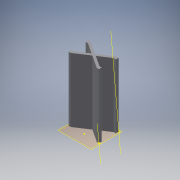
# Autodesk Inventor part: Part3
Saved by Autodesk Inventor 2018 (Build 220112000, 112)
## iProperties
Created: 2019-11-06
Part Number: Part3
Material: Generic
Document SubType Name: Modeling
Designer: bitbots
Density: 1 g/cm^3
Appearance: Default
Author: bitbots
Autodesk Inventor part; units mm, degrees
ref_plane "YZ Plane" through (0, 0, 0) normal (1, 0, 0) x (0, 1, 0)
ref_plane "XZ Plane" through (0, 0, 0) normal (0, 1, 0) x (-1, 0, 0)
ref_plane "XY Plane" through (0, 0, 0) normal (0, 0, 1) x (1, 0, 0)
sketch "Sketch1" plane through (0, 0, 0) normal (0, 0, 1) x (1, 0, 0)
  line L0 (25.85, -1.5771) -> (25.85, -14.5436) construction
  line L1 (25.85, 20.3743) -> (25.85, 33.3441) construction
  line L2 (-26.05, 20.3743) -> (-26.05, 33.3441) construction
  line L3 (-26.05, -1.5771) -> (-26.05, -14.5436) construction
  line L4 (25.85, 20.3743) -> (25.85, 33.3441) construction
  point P0 (0, 0)
ref_plane "Work Plane1" through (25.85, 33.3441, 0) normal (0, 0, 1) x (-1, 0, 0)
sketch "Sketch4" plane through (25.85, 33.3441, 0) normal (0, 0, 1) x (-1, 0, 0)
  line L0 (65.2627, -3.6865) -> (0, -3.6865) construction
  line L1 (55.9, 41.8613) -> (55.9, -3.6865) construction
  line L2 (55.9, -3.6865) -> (0, -3.6865) construction
  line L3 (0, 34.4434) -> (51.9, 0.3135) construction
  line L4 (51.9, 34.4434) -> (0, 0.3135) construction
  line L5 (50.8011, 36.1145) -> (-1.0989, 1.9846) construction
  line L6 (52.9989, 32.7724) -> (1.0989, -1.3575) construction
  line L7 (1.0989, 36.1145) -> (52.9989, 1.9846) construction
  line L8 (-1.0989, 32.7724) -> (50.8011, -1.3575) construction
  line L9 (0, 0.3135) -> (51.9, 0.3135) construction
  line L10 (51.9, 0.3135) -> (51.9, 34.4434) construction
  line L11 (51.9, 34.4434) -> (0, 34.4434) construction
  line L12 (0, 34.4434) -> (0, 0.3135) construction
  line L13 (0, 34.4434) -> (0, 29.4434) construction
  line L14 (0, 34.4434) -> (5, 34.4434) construction
  line L15 (0, 29.4434) -> (3.9633, 29.4434)
  line L16 (0, 0.3135) -> (0, 5.3135) construction
  line L17 (0, 0.3135) -> (5, 0.3135) construction
  line L18 (51.9, 0.3135) -> (51.9, 5.3135) construction
  line L19 (51.9, 0.3135) -> (56.9, 0.3135) construction
  line L20 (51.9, 34.4434) -> (51.9, 29.4434) construction
  line L21 (51.9, 34.4434) -> (56.9, 34.4434) construction
  line L22 (51.9, 29.4434) -> (47.9367, 29.4434)
  line L23 (3.9633, 5.3135) -> (22.31, 17.3785)
  line L24 (47.9367, 5.3135) -> (29.59, 17.3785)
  line L25 (47.9367, 29.4434) -> (29.59, 17.3785)
  line L26 (3.64, 34.4434) -> (25.95, 19.7722)
  line L27 (25.95, 19.7722) -> (48.26, 34.4434)
  line L28 (3.64, 0.3135) -> (25.95, 14.9848)
  line L29 (48.26, 0.3135) -> (25.95, 14.9848)
  line L30 (22.31, 17.3785) -> (3.9633, 29.4434)
  line L31 (51.9, 5.3135) -> (51.9, 0.3135)
  line L32 (51.9, 29.4434) -> (51.9, 34.4434)
  line L33 (0, 5.3135) -> (3.9633, 5.3135)
  line L34 (51.9, 5.3135) -> (47.9367, 5.3135)
  line L35 (51.9, 34.4434) -> (48.26, 34.4434)
  line L36 (0, 34.4434) -> (3.64, 34.4434)
  line L37 (0, 34.4434) -> (0, 29.4434)
  line L38 (3.64, 0.3135) -> (0, 0.3135)
  line L39 (48.26, 0.3135) -> (51.9, 0.3135)
  line L40 (0, 0.3135) -> (0, 5.3135)
  point P0 (25.85, 33.3441)
  point P1 (25.95, 17.3785)
  dimension "d17" = 2
  dimension "d18" = 2
  dimension "d19" = 2
  dimension "d20" = 2
  dimension "d21" = 5
  dimension "d22" = 90
  dimension "d23" = 5
  dimension "d24" = 90
  dimension "d25" = 5
  dimension "d26" = 90
  dimension "d27" = 5
  dimension "d28" = 90
  constraints: 82 end point, 22 point on line, 14 collinear, 7 parallel, 7 perpendicular, 6 horizontal
  measures "d17" distance between parallel lines of L4 L5
  measures "d18" distance between parallel lines of L4 L6
  measures "d19" distance between parallel lines of L3 L7
  measures "d20" distance between parallel lines of L3 L8
  measures "d21" distance of L11.end L13.end
  measures "d22" angle of L13 L14
  measures "d23" distance of L4.end L16.end
  measures "d24" angle of L17 L16
  measures "d25" distance of L9.end L18.end
  measures "d26" angle of L19 L18
  measures "d27" distance of L4.start L20.end
  measures "d28" angle of L20 L21
extrude "Extrusion1" add sketch "Sketch4" along normal blind 110
body "Solid1"
